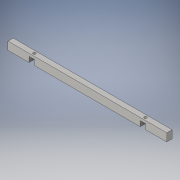
# Autodesk Inventor part: Rack Side
Saved by Autodesk Inventor 2016 (Build 200138000, 138)
## iProperties
Created: 2016-04-12
Part Number: Rack Side
Material: Generic
Document SubType Name: Modeling
Designer: Andrea
Density: 1 g/cm^3
Appearance: Default
Author: Andrea
Autodesk Inventor part; units mm, degrees
ref_plane "YZ Plane" through (0, 0, 0) normal (1, 0, 0) x (0, 1, 0)
ref_plane "XZ Plane" through (0, 0, 0) normal (0, 1, 0) x (-1, 0, 0)
ref_plane "XY Plane" through (0, 0, 0) normal (0, 0, 1) x (1, 0, 0)
sketch "Sketch1" plane through (0, 0, 0) normal (0, 1, 0) x (-1, 0, 0)
  line L0 (0, 0) -> (381, 0)
  line L1 (381, 0) -> (381, -12.7)
  line L2 (381, -12.7) -> (0, -12.7)
  line L3 (0, -12.7) -> (0, 0)
  dimension "d0" = 381
  dimension "d1" = 12.7
  constraints: 8 end point, 2 parallel, 1 horizontal, 1 perpendicular
  measures "d0" distance of L1.end L2.end
  measures "d1" distance of L0.end L1.end
extrude "Extrusion1" add sketch "Sketch1" along normal blind 19.05
sketch "Sketch2" plane through (0, 0, 0) normal (0, -1, 0) x (1, 0, 0)
  line L0 (-63.5, 0) -> (-50.8, 0)
  line L1 (-50.8, 0) -> (-50.8, -12.7)
  line L2 (-50.8, -12.7) -> (-63.5, -12.7)
  line L3 (-63.5, -12.7) -> (-63.5, 0)
  line L4 (0, -12.7) -> (0, 0) projected
  line L5 (-330.2, 0) -> (-317.5, 0)
  line L6 (-317.5, 0) -> (-317.5, -12.7)
  line L7 (-317.5, -12.7) -> (-330.2, -12.7)
  line L8 (-330.2, -12.7) -> (-330.2, 0)
  dimension "d4" = 12.7
  dimension "d5" = 12.7
  dimension "d6" = 50.8
  dimension "d7" = 12.7
  dimension "d8" = 12.7
  dimension "d9" = 330.2
  constraints: 16 end point, 4 parallel, 2 horizontal, 2 perpendicular
  measures "d4" distance of L1.end L2.end
  measures "d5" distance of L0.end L1.end
  measures "d6" distance between parallel lines of L1 L4
  measures "d7" distance of L6.end L7.end
  measures "d8" distance of L5.end L6.end
  measures "d9" distance between parallel lines of L4 L8
extrude "Extrusion2" cut sketch "Sketch2" against normal blind 12.7
sketch "Sketch3" plane through (0, 19.05, 0) normal (0, 1, 0) x (1, 0, 0)
  circle A0 centre (-57.15, 6.35) radius 3.175
  line L0 (0, 0) -> (0, 12.7) projected
  line L1 (0, 12.7) -> (-381, 12.7) projected
  circle A1 centre (-323.85, 6.35) radius 3.175
  dimension "d12" = 6.35
  dimension "d13" = 57.15
  dimension "d15" = 6.35
  dimension "d16" = 6.35
  dimension "d17" = 323.85
  constraints: 2 centre point
  measures "d12" diameter of A0
  measures "d13" distance from line of L0 A0.centre
  measures "d15" distance from line of L1 A0.centre
  measures "d16" diameter of A1
  measures "d17" distance from line of L0 A1.centre
hole "Hole1" at (-323.85, 19.05, -6.35) at (-57.15, 19.05, -6.35) direction (0, -1, 0) diameter 6.35 end through all
body "Solid1"
